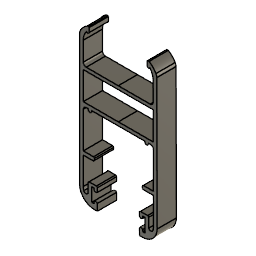
CercoDobleVidrio (Autodesk Fusion 360 design; units mm, degrees)
part number: 2025-12-27-23-45-21-865
Autodesk Fusion 360 part; units mm, degrees
note: some values were not read from the file. Set by a fixed rule: which sketch regions a step uses.
sketch "Boceto2" plane through (0, 0, 0) normal (0, 1, 0) x (1, 0, 0)
  line L0 (7.5, 0) -> (9.2213, 0)
  line L1 (0, -73.2) -> (0, -7.5)
  arc A0 (7.5, 0) -> (0, -7.5) centre (7.5, -7.5) ccw
  line L2 (7.5, -3.5523) -> (7.5, -2.6)
  line L3 (7.5, -2.6) -> (6.3, -2.6)
  line L4 (6.3, -2.6) -> (6.3, -9.6)
  line L5 (6.3, -9.6) -> (7.5, -9.6)
  line L6 (7.5, -9.6) -> (7.5, -8.5)
  line L7 (9.2213, -8.5) -> (9.2213, -10.6)
  line L8 (8.7213, -11.1) -> (4.9, -11.1)
  line L9 (4.4, -10.6) -> (4.4, -5.7)
  arc A1 (4.4, -5.7) -> (2.8546, -5.0381) centre (3.3076, -6.1153) ccw
  arc A2 (4.4, -5.7) -> (2.1854, -5.7893) centre (3.3076, -6.1153) ccw
  arc A3 (2.1854, -5.7893) -> (1.9172, -7.5) centre (7.5062, -7.5) ccw
  arc A4 (9.2213, -8.5) -> (7.5, -8.5) centre (8.3607, -9.2707) ccw
  arc A5 (7.5, -3.5523) -> (9.2213, -3.5523) centre (8.3607, -3.072) ccw
  line L10 (9.2213, -3.5523) -> (9.2213, 0)
  line L11 (20.1126, -1.9172) -> (20.115, -1.9172)
  line L12 (1.9172, -21.6025) -> (7.2, -21.6025)
  line L13 (7.7, -22.1025) -> (7.7, -23)
  line L14 (7.2, -23.5) -> (1.9172, -23.5)
  line L15 (1.9172, -45.6046) -> (20.0634, -45.6046)
  line L16 (20.0634, -43.7426) -> (20.0634, -43.7426)
  line L17 (20.036, -60.0002) -> (20.036, -60.0234)
  line L18 (20.036, -61.8138) -> (3.4172, -61.8138)
  line L19 (1.9172, -21.6025) -> (1.9172, -7.5)
  arc A6 (7.2, -23.5) -> (7.7, -23) centre (7.2, -23) ccw
  arc A7 (7.7, -22.1025) -> (7.2, -21.6025) centre (7.2, -22.1025) ccw
  line L20 (1.9172, -42.2426) -> (1.9172, -23.5)
  arc A8 (1.9172, -42.2426) -> (3.4172, -43.7426) centre (3.4172, -42.2426) ccw
  line L21 (6.2895, -43.7426) -> (6.2895, -43.415)
  line L22 (4.4317, -43.415) -> (4.4317, -43.7426)
  arc A9 (6.2895, -43.415) -> (4.4317, -43.415) centre (5.3606, -43.415) ccw
  line L23 (20.0634, -43.7426) -> (6.2895, -43.7426)
  line L24 (4.4317, -43.7426) -> (3.4172, -43.7426)
  line L25 (1.9172, -73.2) -> (1.9172, -63.3138)
  line L26 (1.9172, -60.0002) -> (1.9172, -45.6046)
  arc A10 (3.4172, -61.8138) -> (1.9172, -63.3138) centre (3.4172, -63.3138) ccw
  arc A11 (4.4, -10.6) -> (4.9, -11.1) centre (4.9, -10.6) ccw
  arc A12 (8.7213, -11.1) -> (9.2213, -10.6) centre (8.7213, -10.6) ccw
  line L27 (32.4735, -22.1342) -> (32.4712, -23.0317)
  line L28 (35.8029, -10.6401) -> (35.8154, -5.7401)
  arc A13 (36.701, -43.7851) -> (38.2048, -42.289) centre (36.7048, -42.2851) ccw
  line L29 (38.1594, -60.0465) -> (38.1962, -45.651)
  line L30 (33.8286, -43.7778) -> (33.8295, -43.4502)
  arc A14 (35.6873, -43.4549) -> (33.8295, -43.4502) centre (34.7584, -43.4526) ccw
  line L31 (32.7209, -3.5846) -> (32.7233, -2.6322)
  line L32 (35.6864, -43.7825) -> (36.701, -43.7851)
  line L33 (32.9699, -23.5329) -> (38.2527, -23.5464)
  line L34 (40.0429, -73.2512) -> (40.2108, -7.5514)
  line L35 (38.2048, -42.289) -> (38.2527, -23.5464)
  arc A15 (32.4712, -23.0317) -> (32.9699, -23.5329) centre (32.9712, -23.0329) ccw
  line L36 (35.6873, -43.4549) -> (35.6864, -43.7825)
  arc A16 (37.3625, -5.0822) -> (35.8154, -5.7401) centre (36.9067, -6.1583) ccw
  line L37 (30.9869, -8.5278) -> (30.9816, -10.6278)
  arc A17 (38.2936, -7.5465) -> (38.0298, -5.8351) centre (32.7046, -7.5322) ccw
  line L38 (32.73, -0.0322) -> (31.0086, -0.0278)
  arc A18 (40.2108, -7.5514) -> (32.73, -0.0322) centre (32.7108, -7.5322) ccw
  arc A19 (35.3016, -11.1388) -> (35.8029, -10.6401) centre (35.3029, -10.6388) ccw
  arc A20 (32.9748, -21.6355) -> (32.4735, -22.1342) centre (32.9735, -22.1355) ccw
  line L39 (32.7054, -9.6322) -> (32.7082, -8.5322)
  arc A21 (30.9816, -10.6278) -> (31.4803, -11.1291) centre (31.4816, -10.6291) ccw
  line L40 (33.9233, -2.6353) -> (33.9054, -9.6353)
  arc A22 (38.0298, -5.8351) -> (35.8154, -5.7401) centre (36.9067, -6.1583) ccw
  arc A23 (38.151, -63.3601) -> (36.6548, -61.8563) centre (36.651, -63.3563) ccw
  arc A24 (30.9996, -3.5802) -> (32.7209, -3.5846) centre (31.8615, -3.102) ccw
  line L41 (30.9996, -3.5802) -> (31.0086, -0.0278)
  line L42 (38.1257, -73.2463) -> (38.151, -63.3601)
  line L43 (38.2576, -21.649) -> (38.2936, -7.5465)
  line L44 (31.4803, -11.1291) -> (35.3016, -11.1388)
  line L45 (32.7233, -2.6322) -> (33.9233, -2.6353)
  line L46 (33.9054, -9.6353) -> (32.7054, -9.6322)
  arc A25 (32.7082, -8.5322) -> (30.9869, -8.5278) centre (31.8456, -9.3007) ccw
  line L47 (38.2576, -21.649) -> (32.9748, -21.6355)
  line L48 (20.0548, -43.7426) -> (33.8286, -43.7778)
  line L49 (38.1962, -45.651) -> (20.05, -45.6046)
  line L50 (20.036, -61.8138) -> (36.6548, -61.8563)
  line L51 (1.9172, -60.0002) -> (38.1594, -60.0465)
  line L52 (20.036, -61.8138) -> (20.0119, -80.7) construction
  line L53 (20.115, 0) -> (20.0591, -43.7426) construction
  line L54 (20.0567, -45.6046) -> (20.0383, -60.0234) construction
  line L55 (20.0119, -80.7) -> (5.0119, -80.7) construction
  line L56 (5.0119, -80.45) -> (5.0119, -78.1977)
  arc A26 (5.0119, -78.1977) -> (3.6157, -77.9747) centre (4.2942, -78.2091) ccw
  arc A27 (1.9172, -73.2) -> (3.6157, -77.9747) centre (9.4774, -73.2) ccw
  line L57 (4.7619, -80.7) -> (4, -80.7)
  line L58 (0, -73.2) -> (0, -75.4021)
  arc A28 (0.432, -77.0212) -> (4, -80.7) centre (9.4618, -71.8331) ccw
  arc A29 (4.7619, -80.7) -> (5.0119, -80.45) centre (4.7619, -80.45) ccw
  arc A30 (0, -75.4021) -> (0.432, -77.0212) centre (3.25, -75.4021) ccw
  arc A31 (36.415, -78.0166) -> (38.1257, -73.2463) centre (30.5655, -73.2269) ccw
  line L59 (40.0429, -73.2512) -> (40.0372, -75.4532)
  arc A32 (39.6011, -77.0712) -> (40.0372, -75.4532) centre (36.7873, -75.4449) ccw
  arc A33 (36.415, -78.0166) -> (35.0182, -78.2361) centre (35.7359, -78.2493) ccw
  line L60 (35.0125, -80.4883) -> (35.0182, -78.2361)
  arc A34 (35.0125, -80.4883) -> (35.2618, -80.739) centre (35.2625, -80.489) ccw
  arc A35 (36.0237, -80.7409) -> (39.6011, -77.0712) centre (30.5846, -71.8601) ccw
  line L61 (35.2618, -80.739) -> (36.0237, -80.7409)
  point P0 (0, -80.7)
  point P1 (40.2299, -0.0514)
  point P2 (40.2299, -0.0514)
  point P3 (35.0118, -80.7383)
  dimension "d10" = 80.7
  dimension "d14" = 0.5
  dimension "d15" = 1.5
  dimension "d16" = 1.5
  dimension "d17" = 0.5
  dimension "d19" = 15
  dimension "d20" = 0.25
  dimension "d21" = 3.25
  constraint horizontal L0
  constraint vertical L1
  constraint coincident P0 L1
  constraint coincident origin L0
  constraint coincident origin L1
  constraint tangent L0 A0
  constraint tangent L1 A0
  constraint perpendicular L2 L3
  constraint perpendicular L2 L5
  constraint perpendicular L5 L6
  constraint perpendicular L3 L7
  constraint perpendicular L7 L8
  constraint perpendicular L8 L9
  constraint concentric A1 A2
  constraint tangent A3 L25
  constraint coincident L11.start L53
  constraint horizontal L12
  constraint vertical L13
  constraint horizontal L14
  constraint coincident L12.start L25
  constraint horizontal L15
  constraint vertical L16
  constraint horizontal L23
  constraint vertical L17
  constraint horizontal L18
  constraint coincident L18.start L53
  constraint coincident L26.start L25
  constraint collinear L19 L25
  constraint tangent L13 A6
  constraint tangent L14 A6
  constraint tangent L12 A7
  constraint tangent L13 A7
  constraint equal A6 A7
  constraint collinear L20 L25
  constraint tangent A8 L23
  constraint tangent L20 A8
  constraint vertical L21
  constraint vertical L22
  constraint coincident L22.end L23
  constraint collinear L23 L24
  constraint collinear L25 L26
  constraint tangent L18 A10
  constraint tangent L25 A10
  constraint tangent L8 A11
  constraint tangent L9 A11
  constraint tangent L7 A12
  constraint tangent L8 A12
  constraint equal A11 A12
  constraint symmetric origin P2 L53
  constraint symmetric L0.start L38.start L53
  constraint symmetric L1.end L34.end L53
  constraint symmetric A0 A18 L53
  constraint symmetric A3.end A17.start L53
  constraint symmetric A5.end A24.start L53
  constraint symmetric L2.start L31.start L53
  constraint symmetric L2.end L31.end L53
  constraint symmetric L3.end L40.start L53
  constraint symmetric L4.end L40.end L53
  constraint symmetric L5.end L39.start L53
  constraint symmetric L6.end L39.end L53
  constraint symmetric L7.start L37.start L53
  constraint symmetric L9.end L28.end L53
  constraint symmetric A1 A16 L53
  constraint symmetric A1.end A16.start L53
  constraint symmetric A2 A22 L53
  constraint symmetric A2.end A17.end L53
  constraint symmetric A3 A17 L53
  constraint symmetric A4 A25 L53
  constraint symmetric A5 A24 L53
  constraint symmetric L0.end L38.end L53
  constraint symmetric L12.start L43.start L53
  constraint symmetric L14.end L33.end L53
  constraint symmetric L15.start L29.end L53
  constraint symmetric L15.end L49.end L53
  constraint symmetric L16.start L48.start L53
  constraint symmetric L26.start L29.start L53
  constraint symmetric L18.start L50.start L53
  constraint symmetric L13.end L27.end L53
  constraint symmetric L14.start L33.start L53
  constraint symmetric A6 A15 L53
  constraint symmetric L12.end A20.start L53
  constraint symmetric L13.start L27.start L53
  constraint symmetric A7 A20 L53
  constraint symmetric A8.end A13.start L53
  constraint symmetric L20.start A13.end L53
  constraint symmetric A8 A13 L53
  constraint symmetric L22.end L32.start L53
  constraint symmetric L21.start L30.start L53
  constraint symmetric L21.end L30.end L53
  constraint symmetric L22.start A14.start L53
  constraint symmetric A9 A14 L53
  constraint symmetric L18.end A23.end L53
  constraint symmetric L25.end A23.start L53
  constraint symmetric A10 A23 L53
  constraint symmetric L8.end A19.start L53
  constraint symmetric L9.start L28.start L53
  constraint symmetric A11 A19 L53
  constraint symmetric L7.end L37.end L53
  constraint symmetric L8.start A21.end L53
  constraint symmetric A12 A21 L53
  constraint coincident L51 L54.end
  constraint collinear L52 L53
  constraint coincident L51 L17.end
  constraint coincident L23 L53.end
  constraint coincident L15 L54.start
  constraint collinear L53 L54
  constraint coincident L48 L16.start
  constraint perpendicular L55 L56
  constraint tangent L25 A27
  constraint perpendicular L56 L57
  constraint parallel L1 L58
  constraint coincident L55.end L57
  constraint coincident L55.end L56
  constraint tangent L57 A29
  constraint tangent L56 A29
  constraint tangent L58 A30
  constraint tangent A28 A30
  constraint symmetric L1.start L52 L34.start
  constraint symmetric L25.start L52 L42.start
  constraint symmetric L52 L55.end P3
  constraint symmetric L52 L56.end A33.end
  constraint symmetric L52 A26.end A31.start
  constraint symmetric L52 A26 A33
  constraint symmetric L52 A27 A31
  constraint symmetric L52 L57.end A35.start
  constraint symmetric L52 A28 A35
  constraint symmetric L52 L57.start A34.end
  constraint symmetric L52 L56.start L60.start
  constraint symmetric L52 A29 A34
  constraint symmetric L52 L58.end L59.end
  constraint symmetric L52 A28.start A32.start
  constraint symmetric L52 A30 A32
  measures "d10" distance of origin P0
  measures "d14" radius of A6
  measures "d15" radius of A8
  measures "d16" radius of A10
  measures "d17" radius of A11
  measures "d19" distance of L52.end L55.end
  measures "d20" radius of A29
  measures "d21" radius of A30
extrude "Extruir1" add sketch "Boceto2" along normal blind 10
equation "L = 10 mm"
equation "d23 = L"
